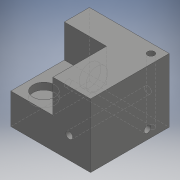
# Autodesk Inventor part: Tophjørne1
Saved by Autodesk Inventor 2018 (Build 220112000, 112)
## iProperties
Created: 2018-01-29
Part Number: Tophjørne1
Material: PC/ABS Plastic
Document SubType Name: Modeling
Designer: MikkelS
Density: 0.357273 g/cm^3
Appearance: Smooth - White
Author: MikkelS
Autodesk Inventor part; units mm, degrees
note: some values were not read from the file. Chosen so that the rebuilt part matches the saved one: direction of "Emboss1".
ref_plane "YZ Plane" through (0, 0, 0) normal (1, 0, 0) x (0, 1, 0)
ref_plane "XZ Plane" through (0, 0, 0) normal (0, 1, 0) x (-1, 0, 0)
ref_plane "XY Plane" through (0, 0, 0) normal (0, 0, 1) x (1, 0, 0)
sketch "Sketch1" plane through (0, 0, 0) normal (0, 0, 1) x (1, 0, 0)
  line L0 (0, 0) -> (0, 69)
  line L1 (0, 69) -> (70, 69)
  line L2 (70, 69) -> (70, 0)
  line L3 (70, 0) -> (0, 0)
  dimension "d0" = 69
  dimension "d1" = 70
  constraints: 8 end point, 3 perpendicular, 1 vertical
  measures "d0" distance of L0.start L0.end
  measures "d1" distance of L0.end L1.end
extrude "Extrusion1" add sketch "Sketch1" along normal blind 56
sketch "Sketch2" plane through (0, 0, 56) normal (0, 0, 1) x (1, 0, 0)
  line L0 (0, 0) -> (37, 0)
  line L1 (37, 0) -> (37, 47)
  line L2 (37, 47) -> (0, 47)
  line L3 (0, 47) -> (0, 0)
  dimension "d4" = 37
  dimension "d5" = 47
  constraints: 8 end point, 3 perpendicular
  measures "d4" distance of L0.start L0.end
  measures "d5" distance of L0.end L1.end
emboss "Emboss1" sketch "Sketch2" operation cut depth 29 direction (0, 0, -1)
sketch "Sketch3" plane through (0, 0, 56) normal (0, 0, 1) x (1, 0, 0)
  circle A0 centre (62, 61) radius 3
  point P0 (0, 0)
  point P1 (70, 69)
  dimension "d10" = 6
  constraints: 1 centre point
  measures "d10" diameter of A0
hole "Hole1" at (62, 61, 56) direction (0, 0, -1) diameter 6 end through all
sketch "Sketch4" plane through (0, 0, 0) normal (-1, 0, 0) x (0, 0, 1)
  circle A0 centre (8, 50) radius 3
  point P0 (0, 69)
  dimension "d20" = 6
  constraints: 1 centre point
  measures "d20" diameter of A0
hole "Hole2" at (0, 50, 8) direction (1, 0, 0) diameter 6 end through all
sketch "Sketch5" plane through (0, 69, 0) normal (0, 1, 0) x (1, 0, 0)
  circle A0 centre (51.2959, -19) radius 3
  dimension "d30" = 6
  constraints: 1 centre point
  measures "d30" diameter of A0
hole "Hole3" at (51.2959, 69, 19) direction (0, -1, 0) diameter 6 end through all
sketch "Sketch6" plane through (0, 47, 27) normal (0, 0, 1) x (1, 0, 0)
  circle A0 centre (14.5, -32.5) radius 9.5
  dimension "d40" = 19
  constraints: 1 centre point
  measures "d40" diameter of A0
hole "Hole4" at (14.5, 14.5, 27) direction (0, 0, -1) diameter 19 depth 6
sketch "Sketch7" plane through (37, 0, 56) normal (-1, 0, 0) x (0, 0, 1)
  circle A0 centre (-14.5, 32.5) radius 9.5
  point P0 (-56, 0)
  point P1 (-29, 47)
  dimension "d50" = 19
  constraints: 1 centre point
  measures "d50" diameter of A0
hole "Hole5" at (37, 32.5, 41.5) direction (1, 0, 0) diameter 19 depth 6
body "Solid1"
